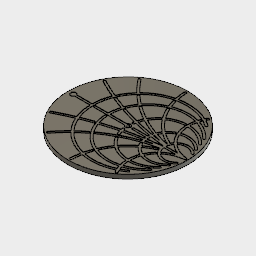
Resizable_Smith_Chart_Complete_7-18 (Autodesk Fusion 360 design; units mm, degrees)
Autodesk Fusion 360 part; units mm, degrees
note: some values were not read from the file. Set by a fixed rule: which sketch regions a step uses.
cylinder "CylinderPrimitive1" add diameter 355.6 height 12.7 placed x (1, 0, 0) y (0, 0, -1) z (0, 1, 0) at (0, 0, 0)
sketch "Smith Chart Overlay" plane through (0, 12.7, 0) normal (0, 1, 0) x (-1, 0, 0)
  circle A0 centre (0, 0) radius 177.8
  circle A1 centre (0, 0) radius 177.8
  line L0 (0, 0) -> (-177.8, 0)
  line L1 (0, 0) -> (-118.5333, 0) construction
  line L2 (0, 0) -> (-88.9, 0)
  line L3 (0, 0) -> (-59.2667, 0)
  circle A2 centre (-118.5333, 0) radius 59.2667 construction
  circle A3 centre (-88.9, 0) radius 88.9 construction
  circle A4 centre (-59.2667, 0) radius 118.5333 construction
  arc A5 (-106.68, -142.24) -> (-177.8, 0) centre (-177.8, -88.9) ccw construction
  line L4 (-177.8, 0) -> (-177.8, -88.9)
  line L5 (-177.8, 0) -> (-177.8, 88.9)
  line L6 (-177.8, 177.8) -> (-177.8, 0)
  line L7 (-177.8, 0) -> (-177.8, -177.8)
  line L8 (-177.8, 0) -> (-177.8, -355.6)
  arc A6 (-177.8, 0) -> (-106.68, 142.24) centre (-177.8, 88.9) ccw construction
  arc A7 (0, -177.8) -> (-177.8, 0) centre (-177.8, -177.8) ccw construction
  arc A8 (-177.8, 0) -> (0, 177.8) centre (-177.8, 177.8) ccw construction
  line L9 (-177.8, 355.6) -> (-177.8, 0)
  arc A9 (106.68, -142.24) -> (-177.8, 0) centre (-177.8, -355.6) ccw construction
  arc A10 (-177.8, 0) -> (106.68, 142.24) centre (-177.8, 355.6) ccw construction
  line L10 (-13.7583, 0) -> (-73.025, 0)
  line L11 (0, 0) -> (-59.2667, 0)
  line L12 (0, 0) -> (-35.56, 0)
  circle A11 centre (-35.56, 0) radius 142.24 construction
  line L13 (-177.8, 0) -> (-177.8, -711.2)
  arc A12 (156.8824, -83.6706) -> (-177.8, 0) centre (-177.8, -711.2) ccw construction
  arc A13 (-177.8, 0) -> (156.8824, 83.6706) centre (-177.8, 711.2) ccw construction
  line L14 (0, 0) -> (-142.24, 0) construction
  circle A14 centre (-142.24, 0) radius 35.56 construction
  line L15 (-35.56, 0) -> (177.8, 0) construction
  line L16 (-142.24, 0) -> (-168.4576, 24.024) construction
  line L17 (-142.24, 0) -> (-152.4, 0) construction
  line L18 (-142.24, 0) -> (-168.4576, -24.024) construction
  line L19 (-142.24, 0) -> (-168.4576, 24.024) construction
  line L20 (-118.5333, 0) -> (-162.2293, 40.04) construction
  line L21 (-118.5333, 0) -> (-149.1382, 0) construction
  arc A15 (-162.2293, -40.04) -> (-162.2293, 40.04) centre (-118.5333, 0) ccw construction
  line L22 (-118.5333, 0) -> (-162.2293, -40.04) construction
  line L23 (-118.5333, 0) -> (-162.2293, 40.04) construction
  line L24 (-88.9, 0) -> (-154.444, -60.06) construction
  line L25 (-88.9, 0) -> (-123.6401, 0) construction
  arc A16 (-154.444, -60.06) -> (-154.444, 60.06) centre (-88.9, 0) ccw construction
  line L26 (-88.9, 0) -> (-154.444, -60.06) construction
  line L27 (-88.9, 0) -> (-154.444, 60.06) construction
  line L28 (-35.56, 0) -> (-117.1455, -116.5162) construction
  line L29 (-35.56, 0) -> (214.1255, 0) construction
  line L30 (-59.2667, 0) -> (59.2667, 0) construction
  arc A17 (52.8595, 38.4432) -> (-92.456, 113.792) centre (-59.2667, 0) ccw
  line L31 (-177.8, -711.2) -> (-177.8, 711.2)
  line L32 (-59.2667, 0) -> (-146.6586, 80.08) construction
  line L33 (-59.2667, 0) -> (75.6719, 0) construction
  arc A18 (-146.6586, -80.08) -> (-146.6586, 80.08) centre (-59.2667, 0) ccw construction
  line L34 (-59.2667, 0) -> (-146.6586, -80.08) construction
  line L35 (-59.2667, 0) -> (-146.6586, 80.08) construction
  arc A19 (-117.1455, -116.5162) -> (-117.1455, 116.5162) centre (-35.56, 0) ccw construction
  line L36 (-35.56, 0) -> (-117.1455, -116.5162) construction
  line L37 (-35.56, 0) -> (-117.1455, 116.5162) construction
  arc A20 (-92.456, 113.792) -> (-97.8899, 127.8562) centre (-177.8, 88.9) ccw
  arc A21 (-60.0841, 9.8097) -> (52.8595, 38.4432) centre (-177.8, 711.2) ccw
  arc A22 (-60.0841, 9.8097) -> (-62.4703, 19.2216) centre (-118.5333, 0) ccw
  arc A23 (-107.3842, 7.0416) -> (-62.4703, 19.2216) centre (-177.8, 355.6) ccw
  arc A24 (-97.8899, -127.8562) -> (106.68, 0) centre (-35.56, 0) ccw
  arc A25 (-95.7385, -54.7077) -> (-116.4897, -24.5241) centre (-177.8, -88.9) ccw
  arc A26 (-92.456, -113.792) -> (-95.7385, -54.7077) centre (-177.8, -88.9) ccw
  arc A27 (-92.456, -113.792) -> (59.2667, 0) centre (-59.2667, 0) ccw
  circle A28 centre (106.68, 0) radius 7.62 construction
  circle A29 centre (59.2667, 0) radius 7.62 construction
  circle A30 centre (52.8595, -38.4432) radius 7.62 construction
  circle A31 centre (95.7385, -54.7077) radius 7.62 construction
  circle A32 centre (67.4414, -98.0966) radius 7.62 construction
  circle A33 centre (35.56, -71.12) radius 7.62 construction
  circle A34 centre (52.8595, 38.4432) radius 7.62 construction
  circle A35 centre (95.7385, 54.7077) radius 7.62 construction
  circle A36 centre (67.4414, 98.0966) radius 7.62 construction
  circle A37 centre (-97.8899, 127.8562) radius 7.62 construction
  circle A38 centre (-88.9, 88.9) radius 7.62 construction
  circle A39 centre (-13.6769, 109.4154) radius 7.62 construction
  circle A40 centre (-92.456, 113.792) radius 7.62 construction
  circle A41 centre (35.56, 71.12) radius 7.62 construction
  circle A42 centre (-2.7354, 21.8831) radius 7.62 construction
  circle A43 centre (-10.4588, 41.8353) radius 7.62 construction
  circle A44 centre (-35.56, 71.12) radius 7.62 construction
  circle A45 centre (0, 0) radius 15.24 construction
  circle A46 centre (-2.7354, -21.8831) radius 7.62 construction
  circle A47 centre (-10.4588, -41.8353) radius 7.62 construction
  circle A48 centre (-35.56, -71.12) radius 7.62 construction
  circle A49 centre (-88.9, -88.9) radius 7.62 construction
  circle A50 centre (-95.7385, -54.7077) radius 7.62 construction
  circle A51 centre (-95.7385, 54.7077) radius 7.62 construction
  circle A52 centre (-59.2667, 0) radius 7.62 construction
  circle A53 centre (-116.4897, -24.5241) radius 7.62 construction
  circle A54 centre (-116.4897, 24.5241) radius 7.62 construction
  circle A55 centre (-71.12, 35.56) radius 7.62 construction
  circle A56 centre (-4.3366, 138.7707) radius 7.62 construction
  circle A57 centre (-71.12, -35.56) radius 7.62 construction
  circle A58 centre (-92.456, -113.792) radius 7.62 construction
  circle A59 centre (-13.6769, -109.4154) radius 7.62 construction
  circle A60 centre (-97.8899, -127.8562) radius 7.62 construction
  circle A61 centre (-4.3366, -138.7707) radius 7.62 construction
  circle A62 centre (156.8824, -83.6706) radius 7.62 construction
  circle A63 centre (106.68, -142.24) radius 7.62 construction
  circle A64 centre (0, -177.8) radius 7.62 construction
  circle A65 centre (-106.68, -142.24) radius 7.62 construction
  circle A66 centre (-106.68, 142.24) radius 7.62 construction
  circle A67 centre (0, 177.8) radius 7.62 construction
  circle A68 centre (106.68, 142.24) radius 7.62 construction
  circle A69 centre (156.8824, 83.6706) radius 7.62 construction
  circle A70 centre (177.8, 0) radius 15.24 construction
  arc A71 (-117.1455, -116.5162) -> (-117.1455, 116.5162) centre (-35.56, 0) ccw
  line L38 (106.68, 0) -> (162.56, 0)
  arc A72 (150.1397, -80.1208) -> (95.7385, -54.7077) centre (-177.8, -711.2) ccw
  arc A73 (102.0429, -136.1933) -> (67.4414, -98.0966) centre (-177.8, -355.6) ccw
  arc A74 (-0.1633, -170.1817) -> (-4.3366, -138.7707) centre (-177.8, -177.8) ccw
  arc A75 (-102.3735, -135.9537) -> (-97.8899, -127.8562) centre (-177.8, -88.9) ccw
  arc A76 (95.7385, 54.7077) -> (150.1397, 80.1208) centre (-177.8, 711.2) ccw
  arc A77 (67.4414, 98.0966) -> (102.0429, 136.1933) centre (-177.8, 355.6) ccw
  arc A78 (-4.3366, 138.7707) -> (-0.1633, 170.1817) centre (-177.8, 177.8) ccw
  arc A79 (-97.8899, 127.8562) -> (-102.3735, 135.9537) centre (-177.8, 88.9) ccw
  arc A80 (-146.6586, -80.08) -> (-92.456, -113.792) centre (-59.2667, 0) ccw
  arc A81 (-111.202, 30.011) -> (-92.456, 113.792) centre (-177.8, 88.9) ccw
  arc A82 (-94.8474, -120.8699) -> (-92.456, -113.792) centre (-177.8, -88.9) ccw
  arc A83 (-6.1682, -131.3741) -> (-13.6769, -109.4154) centre (-177.8, -177.8) ccw
  arc A84 (61.8675, -92.9008) -> (35.56, -71.12) centre (-177.8, -355.6) ccw
  arc A85 (88.689, -51.8146) -> (52.8595, -38.4432) centre (-177.8, -711.2) ccw
  arc A86 (-168.4576, -24.024) -> (-168.4576, 24.024) centre (-142.24, 0) ccw
  arc A87 (-16.7577, -102.446) -> (-109.4154, -13.6769) centre (-177.8, -177.8) ccw
  arc A88 (-88.9076, -51.3308) -> (-60.0841, 9.8097) centre (-118.5333, 0) ccw
  circle A89 centre (-62.4703, 19.2216) radius 7.62 construction
  arc A90 (-62.4703, 19.2216) -> (29.4154, 66.6136) centre (-177.8, 355.6) ccw
  arc A91 (60.0542, 40.9532) -> (95.7385, 54.7077) centre (-177.8, 711.2) ccw
  arc A92 (41.6067, 75.7571) -> (67.4414, 98.0966) centre (-177.8, 355.6) ccw
  arc A93 (-10.8976, 116.5104) -> (-4.3366, 138.7707) centre (-177.8, 177.8) ccw
  line L39 (59.2667, 0) -> (0, 0)
  arc A94 (-1.3063, 15.1839) -> (-2.7354, 21.8831) centre (-88.9, 0) ccw
  arc A95 (59.0217, 7.6161) -> (52.8595, 38.4432) centre (-59.2667, 0) ccw
  line L40 (99.06, 0) -> (59.2667, 0)
  arc A96 (-95.7385, 54.7077) -> (-162.2293, 40.04) centre (-118.5333, 0) ccw
  circle A97 centre (-109.4154, 13.6769) radius 7.62 construction
  arc A98 (-102.446, 16.7577) -> (-13.6769, 109.4154) centre (-177.8, 177.8) ccw
  arc A99 (29.4154, -66.6136) -> (-107.3842, -7.0416) centre (-177.8, -355.6) ccw
  arc A100 (-81.287, -88.5734) -> (-1.3063, -15.1839) centre (-88.9, 0) ccw
  arc A101 (-154.444, -60.06) -> (-88.9, -88.9) centre (-88.9, 0) ccw
  line L41 (-15.24, 0) -> (-59.2667, 0)
  arc A102 (-60.0841, 9.8097) -> (-2.7354, 21.8831) centre (-177.8, 711.2) ccw
  arc A103 (-106.8574, 3.5471) -> (-60.0841, 9.8097) centre (-177.8, 711.2) ccw
  arc A104 (45.6382, -36.0105) -> (-106.8574, -3.5471) centre (-177.8, -711.2) ccw
  arc A105 (-88.9, 88.9) -> (-154.444, 60.06) centre (-88.9, 0) ccw
  arc A106 (-92.456, 113.792) -> (-146.6586, 80.08) centre (-59.2667, 0) ccw
  arc A107 (-65.3999, 26.2559) -> (-95.7385, 54.7077) centre (-118.5333, 0) ccw
  arc A108 (-14.3296, 48.399) -> (-88.9, 88.9) centre (-88.9, 0) ccw
  arc A109 (-2.7354, 21.8831) -> (-7.1644, 34.9643) centre (-88.9, 0) ccw
  circle A110 centre (0, 0) radius 7.62
  circle A111 centre (162.56, 0) radius 7.62
  circle A112 centre (150.1397, 80.1208) radius 3.175
  circle A113 centre (102.0429, 136.1933) radius 3.175
  circle A114 centre (-0.1633, 170.1817) radius 3.175
  circle A115 centre (-102.3735, 135.9537) radius 3.175
  circle A116 centre (150.1397, -80.1208) radius 3.175
  circle A117 centre (102.0429, -136.1933) radius 3.175
  circle A118 centre (-0.1633, -170.1817) radius 3.175
  circle A119 centre (-102.3735, -135.9537) radius 3.175
  circle A120 centre (-117.1455, -116.5162) radius 3.175
  circle A121 centre (-146.6586, -80.08) radius 3.175
  circle A122 centre (-154.444, -60.06) radius 3.175
  circle A123 centre (-168.4576, -24.024) radius 3.175
  circle A124 centre (-168.4576, 24.024) radius 3.175
  circle A125 centre (-162.2293, 40.04) radius 3.175
  circle A126 centre (-154.444, 60.06) radius 3.175
  circle A127 centre (-146.6586, 80.08) radius 3.175
  circle A128 centre (-117.1455, 116.5162) radius 3.175
  circle A129 centre (-14.3296, 48.399) radius 3.175
  circle A130 centre (-7.1644, 34.9643) radius 3.175
  circle A131 centre (-1.3063, 15.1839) radius 3.175
  circle A132 centre (-1.3063, -15.1839) radius 3.175
  circle A133 centre (-15.24, 0) radius 3.175
  circle A134 centre (59.0217, 7.6161) radius 3.175
  circle A135 centre (99.06, 0) radius 3.175
  circle A136 centre (60.0542, 40.9532) radius 3.175
  circle A137 centre (41.6067, 75.7571) radius 3.175
  circle A138 centre (-10.8976, 116.5104) radius 3.175
  circle A139 centre (-65.3999, 26.2559) radius 3.175
  circle A140 centre (-111.202, 30.011) radius 3.175
  circle A141 centre (-102.446, 16.7577) radius 3.175
  arc A142 (-162.2293, -40.04) -> (-95.7385, -54.7077) centre (-118.5333, 0) ccw
  circle A143 centre (-162.2293, -40.04) radius 3.175
  circle A144 centre (-88.9076, -51.3308) radius 3.175
  circle A145 centre (-81.287, -88.5734) radius 3.175
  circle A146 centre (45.6382, -36.0105) radius 3.175
  circle A147 centre (29.4154, -66.6136) radius 3.175
  circle A148 centre (-16.7577, -102.446) radius 3.175
  circle A149 centre (88.689, -51.8146) radius 3.175
  circle A150 centre (61.8675, -92.9008) radius 3.175
  circle A151 centre (-6.1682, -131.3741) radius 3.175
  circle A152 centre (-94.8474, -120.8699) radius 3.175
  circle A153 centre (29.4154, 66.6136) radius 3.175
  circle A154 centre (0, 0) radius 3.81
  circle A155 centre (-177.8, 0) radius 7.62 construction
  arc A156 (-170.187, 0.3266) -> (-116.4897, 24.5241) centre (-177.8, 88.9) ccw
  arc A157 (-116.4897, -24.5241) -> (-170.187, -0.3266) centre (-177.8, -88.9) ccw
  line L42 (-106.68, 0) -> (-170.18, 0)
  circle A158 centre (-170.18, 0) radius 3.501
  point P0 (-13.6769, 109.4154)
  point P1 (95.7385, 54.7077)
  point P2 (67.4414, 98.0966)
  point P3 (-97.8899, 127.8562)
  point P4 (106.68, 0)
  point P5 (95.7385, -54.7077)
  point P6 (67.4414, -98.0966)
  point P7 (-4.3366, -138.7707)
  point P8 (-97.8899, -127.8562)
  point P9 (-92.456, 113.792)
  point P10 (35.56, 71.12)
  point P11 (52.8595, 38.4432)
  point P12 (52.8595, -38.4432)
  point P13 (35.56, -71.12)
  point P14 (-13.6769, -109.4154)
  point P15 (-92.456, -113.792)
  point P16 (-35.56, 71.12)
  point P17 (-88.9, 88.9)
  point P18 (-10.4588, 41.8353)
  point P19 (-2.7354, -21.8831)
  point P20 (-88.9, -88.9)
  point P21 (-10.4588, -41.8353)
  point P22 (-35.56, -71.12)
  point P23 (-154.444, -60.06)
  point P24 (-2.7354, 21.8831)
  point P25 (-95.7385, 54.7077)
  point P26 (-71.12, 35.56)
  point P27 (-62.4703, 19.2216)
  point P28 (-60.0841, -9.8097)
  point P29 (-62.4703, -19.2216)
  point P30 (-71.12, -35.56)
  point P31 (-95.7385, -54.7077)
  point P32 (-60.0841, 9.8097)
  point P33 (-116.4897, 24.5241)
  point P34 (-177.8, 0)
  point P35 (-178.44, 0.0003)
  point P36 (106.68, 142.24)
  point P37 (0, 177.8)
  point P38 (156.8824, 83.6706)
  point P39 (156.8824, -83.6706)
  point P40 (177.8, 0)
  point P41 (106.68, -142.24)
  point P42 (0, -177.8)
  point P43 (59.2667, 0)
  point P44 (-177.8, -0.0001)
  point P45 (45.6382, 36.0105)
  point P46 (55.0978, 31.1594)
  point P47 (60.0542, 40.9532)
  point P48 (50.1577, 45.5682)
  point P49 (98.4798, 47.5979)
  point P50 (102.7565, 57.6761)
  point P51 (88.689, 51.8146)
  point P52 (92.6203, 61.6605)
  point P53 (99.06, 0)
  point P54 (106.4759, -7.6173)
  point P55 (106.4759, 7.6173)
  point P56 (59.0217, -7.6161)
  point P57 (51.6467, 0)
  point P58 (66.8867, 0)
  point P59 (88.689, -51.8146)
  point P60 (92.6203, -61.6605)
  point P61 (102.7565, -57.6761)
  point P62 (39.9337, -64.8802)
  point P63 (30.7944, -77.0659)
  point P64 (41.6067, -75.7571)
  point P65 (29.4154, -66.6136)
  point P66 (72.5469, -92.4398)
  point P67 (62.0403, -103.4717)
  point P68 (72.9027, -103.4105)
  point P69 (61.8675, -92.9008)
  point P70 (61.8675, 92.9008)
  point P71 (62.0403, 103.4717)
  point P72 (72.5469, 92.4398)
  point P73 (72.9027, 103.4105)
  point P74 (-10.8976, 116.5104)
  point P75 (-16.7577, 102.446)
  point P76 (-6.7409, 106.26)
  point P77 (-6.7409, 106.26)
  point P78 (-85.076, 115.6894)
  point P79 (-90.6379, 106.3921)
  point P80 (-94.9012, 121.009)
  point P81 (-99.6988, 111.4244)
  point P82 (-40.2616, 65.1234)
  point P83 (-31.1197, 77.3126)
  point P84 (-29.6655, 66.2909)
  point P85 (-41.8463, 75.4265)
  point P86 (-81.287, 88.5734)
  point P87 (-89.2266, 81.287)
  point P88 (-89.2266, 96.513)
  point P89 (-96.513, 88.5734)
  point P90 (-17.2204, 38.3217)
  point P91 (-7.1644, 34.9643)
  point P92 (-3.7741, 45.493)
  point P93 (-14.3296, 48.399)
  point P94 (114.3, 0)
  point P95 (98.4798, -47.5979)
  point P96 (59.0217, -7.6161)
  point P97 (60.0542, -40.9532)
  point P98 (50.1577, -45.5682)
  point P99 (45.6382, -36.0105)
  point P100 (55.0978, -31.1594)
  point P101 (-31.1197, -77.3126)
  point P102 (-41.8463, -75.4265)
  point P103 (-29.6655, -66.2909)
  point P104 (-40.2616, -65.1234)
  point P105 (-89.2266, -81.287)
  point P106 (-89.2266, -96.513)
  point P107 (-81.287, -88.5734)
  point P108 (-96.513, -88.5734)
  point P109 (-93.1118, -61.8607)
  point P110 (-98.968, -47.8059)
  point P111 (-102.9462, -57.1802)
  point P112 (-102.9462, -57.1802)
  point P113 (-111.8559, 18.4749)
  point P114 (-111.202, 30.011)
  point P115 (-122.3058, 29.4473)
  point P116 (-122.2277, 19.5103)
  point P117 (-98.968, 47.8059)
  point P118 (-102.9462, 57.1802)
  point P119 (-88.9076, 51.3308)
  point P120 (-93.1118, 61.8607)
  point P121 (-4.3366, 138.7707)
  point P122 (-66.9493, 29.1827)
  point P123 (-77.3126, 31.1197)
  point P124 (-76.0744, 41.3495)
  point P125 (-65.1234, 40.2616)
  point P126 (-104.6474, 124.3348)
  point P127 (-94.8474, 120.8699)
  point P128 (-101.5195, 134.5562)
  point P129 (-90.9535, 131.0106)
  point P130 (-17.2204, -38.3217)
  point P131 (-14.3296, -48.399)
  point P132 (-3.7741, -45.493)
  point P133 (-7.1644, -34.9643)
  point P134 (-4.9259, -29.1814)
  point P135 (4.64, -23.7983)
  point P136 (-1.1779, -14.4239)
  point P137 (-10.1309, -20.047)
  point P138 (-15.24, 0)
  point P139 (-1.3063, -15.1839)
  point P140 (15.24, 0)
  point P141 (-1.3063, 15.1839)
  point P142 (-1.1779, 14.4239)
  point P143 (4.64, 23.7983)
  point P144 (-10.1309, 20.047)
  point P145 (-4.9259, 29.1814)
  point P146 (3.0501, 136.8995)
  point P147 (-6.1682, 131.3741)
  point P148 (-11.8129, 140.2437)
  point P149 (-2.8236, 146.239)
  point P150 (-65.1234, -40.2616)
  point P151 (-76.0744, -41.3495)
  point P152 (-77.3126, -31.1197)
  point P153 (-51.6467, 0)
  point P154 (-59.7565, 7.6042)
  point P155 (-59.7565, 7.6042)
  point P156 (-66.8867, 0)
  point P157 (3.0501, -136.8995)
  point P158 (-2.8236, -146.239)
  point P159 (-6.1682, -131.3741)
  point P160 (-11.8129, -140.2437)
  point P161 (-20.8013, -112.1186)
  point P162 (-10.8976, -116.5104)
  point P163 (-6.7409, -106.26)
  point P164 (-16.7577, -102.446)
  point P165 (-192.3786, -267.9595)
  point P166 (-210, -290)
  point P167 (-225, -285)
  point P168 (-220, -260)
  point P169 (-180, -255)
  point P170 (-215, -245)
  point P171 (-185, -235)
  point P172 (-200, -225)
  point P173 (162.56, 0)
  point P174 (150.1397, 80.1208)
  point P175 (150.1397, -80.1208)
  point P176 (102.0429, -136.1933)
  point P177 (-0.1633, -170.1817)
  point P178 (-102.3735, -135.9537)
  point P179 (-102.3735, 135.9537)
  point P180 (-0.1633, 170.1817)
  point P181 (102.0429, 136.1933)
  point P182 (59.0217, 7.6161)
  point P183 (-104.6474, -124.3348)
  point P184 (-101.5195, -134.5562)
  point P185 (-90.9535, -131.0106)
  point P186 (-94.8474, -120.8699)
  point P187 (-88.9076, -51.3308)
  point P188 (-66.9493, -29.1827)
  point P189 (-122.2277, -19.5103)
  point P190 (-122.3058, -29.4473)
  point P191 (-111.202, -30.011)
  point P192 (-111.8559, -18.4749)
  point P193 (-109.4154, -13.6769)
  point P194 (-107.3842, -7.0416)
  point P195 (-60.4674, 11.8696)
  point P196 (-69.7044, 16.8276)
  point P197 (-65.3999, 26.2559)
  point P198 (-55.2891, 21.7701)
  point P199 (29.4154, 66.6136)
  point P200 (39.9337, 64.8802)
  point P201 (41.6067, 75.7571)
  point P202 (30.7944, 77.0659)
  point P203 (-109.4154, 13.6769)
  point P204 (-116.5104, 10.8976)
  point P205 (-107.2551, 6.3696)
  point P206 (-102.446, 16.7577)
  point P207 (-113.0829, 20.3563)
  point P208 (-106.8574, 3.5471)
  point P209 (-107.3842, 7.0416)
  point P210 (-106.8574, -3.5471)
  point P211 (-170.18, 0)
  point P212 (-170.187, 0.3266)
  point P213 (-170.187, -0.3266)
  point P214 (-106.68, 0)
  dimension "d6" = 355.6
  dimension "d7" = 177.8
  dimension "d8" = 118.5333
  dimension "d11" = 59.2667
  dimension "d12" = 118.5333
  dimension "d13" = 177.8
  dimension "d14" = 237.0667
  dimension "d15" = 88.9
  dimension "d17" = 88.9
  dimension "d18" = 88.9
  dimension "d19" = 177.8
  dimension "d20" = 177.8
  dimension "d21" = 355.6
  dimension "d22" = 88.9
  dimension "d23" = 177.8
  dimension "d24" = 355.6
  dimension "d25" = 59.2667
  dimension "d26" = 59.2667
  dimension "d31" = 35.56
  dimension "d32" = 284.48
  dimension "d33" = 711.2
  dimension "d34" = 711.2
  dimension "d35" = 142.24
  dimension "d36" = 71.12
  dimension "d54" = 137.5
  dimension "d55" = 85
  dimension "d56" = 137.5
  dimension "d57" = 85
  dimension "d58" = 137.5
  dimension "d59" = 85
  dimension "d60" = 125
  dimension "d64" = 118.5333
  dimension "d65" = 1422.4
  dimension "d68" = 137.5
  dimension "d69" = 85
  dimension "d70" = 110
  dimension "d79" = 15.24
  dimension "d80" = 15.24
  dimension "d81" = 15.24
  dimension "d82" = 15.24
  dimension "d83" = 15.24
  dimension "d84" = 15.24
  dimension "d85" = 15.24
  dimension "d86" = 15.24
  dimension "d87" = 15.24
  dimension "d88" = 15.24
  dimension "d89" = 15.24
  dimension "d90" = 15.24
  dimension "d91" = 15.24
  dimension "d92" = 15.24
  dimension "d93" = 15.24
  dimension "d94" = 15.24
  dimension "d95" = 15.24
  dimension "d96" = 30.48
  dimension "d97" = 15.24
  dimension "d98" = 15.24
  dimension "d99" = 15.24
  dimension "d100" = 15.24
  dimension "d101" = 15.24
  dimension "d102" = 15.24
  dimension "d103" = 15.24
  dimension "d104" = 15.24
  dimension "d105" = 15.24
  dimension "d106" = 15.24
  dimension "d107" = 15.24
  dimension "d108" = 15.24
  dimension "d109" = 15.24
  dimension "d110" = 15.24
  dimension "d111" = 15.24
  dimension "d112" = 15.24
  dimension "d113" = 15.24
  dimension "d114" = 15.24
  dimension "d115" = 15.24
  dimension "d116" = 15.24
  dimension "d117" = 15.24
  dimension "d118" = 15.24
  dimension "d119" = 15.24
  dimension "d120" = 15.24
  dimension "d121" = 30.48
  dimension "d251" = 15.24
  dimension "d288" = 15.24
  dimension "d341" = 15.24
  dimension "d342" = 15.24
  dimension "d348" = 6.35
  dimension "d349" = 6.35
  dimension "d350" = 6.35
  dimension "d351" = 6.35
  dimension "d352" = 6.35
  dimension "d353" = 6.35
  dimension "d354" = 6.35
  dimension "d355" = 6.35
  dimension "d356" = 6.35
  dimension "d357" = 6.35
  dimension "d358" = 6.35
  dimension "d359" = 6.35
  dimension "d360" = 6.35
  dimension "d361" = 6.35
  dimension "d362" = 6.35
  dimension "d363" = 6.35
  dimension "d364" = 6.35
  dimension "d365" = 6.35
  dimension "d366" = 6.35
  dimension "d367" = 6.35
  dimension "d368" = 6.35
  dimension "d369" = 6.35
  dimension "d370" = 6.35
  dimension "d371" = 6.35
  dimension "d372" = 6.35
  dimension "d373" = 6.35
  dimension "d374" = 6.35
  dimension "d375" = 6.35
  dimension "d376" = 6.35
  dimension "d377" = 6.35
  dimension "d382" = 6.35
  dimension "d383" = 6.35
  dimension "d384" = 6.35
  dimension "d385" = 6.35
  dimension "d386" = 6.35
  dimension "d387" = 6.35
  dimension "d388" = 6.35
  dimension "d389" = 6.35
  dimension "d390" = 6.35
  dimension "d391" = 6.35
  dimension "d405" = 6.35
  dimension "d412" = 7.62
  dimension "d416" = 15.24
  dimension "d429" = 7.002
  measures "d6" diameter of A1
  measures "d7" distance of A0.centre P34
  measures "d8" distance of A0.centre L1.end
  measures "d11" distance of A0.centre L3.end
  measures "d12" diameter of A2
  measures "d13" diameter of A3
  measures "d14" diameter of A4
  measures "d15" radius of A5
  measures "d17" distance of P34 A5.centre
  measures "d18" distance of P34 L5.end
  measures "d19" distance of L6.start P34
  measures "d20" distance of P34 L7.end
  measures "d21" distance of P34 L8.end
  measures "d22" radius of A6
  measures "d23" radius of A7
  measures "d24" distance of L9.start L0.end
  measures "d25" distance of L10.end L10.start
  measures "d26" distance of L3.end A0.centre
  measures "d31" distance of A0.centre L12.end
  measures "d32" diameter of A11
  measures "d33" distance of P34 L13.end
  measures "d34" distance of P34 A13.centre
  measures "d35" distance of A0.centre L14.end
  measures "d36" diameter of A14
  measures "d54" angle of L16 L17
  measures "d55" angle of L18 L19
  measures "d56" angle of L20 L21
  measures "d57" angle of L22 L23
  measures "d58" angle of L24 L25
  measures "d59" angle of L26 L27
  measures "d60" angle of L28 L29
  measures "d64" radius of A17
  measures "d65" distance of L13.end A13.centre
  measures "d68" angle of L32 L33
  measures "d69" angle of L34 L35
  measures "d70" angle of L36 L37
  measures "d79" diameter of A28
  measures "d80" diameter of A29
  measures "d81" diameter of A30
  measures "d82" diameter of A31
  measures "d83" diameter of A32
  measures "d84" diameter of A33
  measures "d85" diameter of A34
  measures "d86" diameter of A35
  measures "d87" diameter of A36
  measures "d88" diameter of A37
  measures "d89" diameter of A38
  measures "d90" diameter of A39
  measures "d91" diameter of A40
  measures "d92" diameter of A41
  measures "d93" diameter of A42
  measures "d94" diameter of A43
  measures "d95" diameter of A44
  measures "d96" diameter of A45
  measures "d97" diameter of A46
  measures "d98" diameter of A47
  measures "d99" diameter of A48
  measures "d100" diameter of A49
  measures "d101" diameter of A50
  measures "d102" diameter of A51
  measures "d103" diameter of A52
  measures "d104" diameter of A53
  measures "d105" diameter of A54
  measures "d106" diameter of A55
  measures "d107" diameter of A56
  measures "d108" diameter of A57
  measures "d109" diameter of A58
  measures "d110" diameter of A59
  measures "d111" diameter of A60
  measures "d112" diameter of A61
  measures "d113" diameter of A62
  measures "d114" diameter of A63
  measures "d115" diameter of A64
  measures "d116" diameter of A65
  measures "d117" diameter of A66
  measures "d118" diameter of A67
  measures "d119" diameter of A68
  measures "d120" diameter of A69
  measures "d121" diameter of A70
  measures "d251" diameter of A89
  measures "d288" diameter of A97
  measures "d341" diameter of A110
  measures "d342" diameter of A111
  measures "d348" diameter of A112
  measures "d349" diameter of A113
  measures "d350" diameter of A114
  measures "d351" diameter of A115
  measures "d352" diameter of A116
  measures "d353" diameter of A117
  measures "d354" diameter of A118
  measures "d355" diameter of A119
  measures "d356" diameter of A120
  measures "d357" diameter of A121
  measures "d358" diameter of A122
  measures "d359" diameter of A123
  measures "d360" diameter of A124
  measures "d361" diameter of A125
  measures "d362" diameter of A126
  measures "d363" diameter of A127
  measures "d364" diameter of A128
  measures "d365" diameter of A129
  measures "d366" diameter of A130
  measures "d367" diameter of A131
  measures "d368" diameter of A132
  measures "d369" diameter of A133
  measures "d370" diameter of A134
  measures "d371" diameter of A135
  measures "d372" diameter of A136
  measures "d373" diameter of A137
  measures "d374" diameter of A138
  measures "d375" diameter of A139
  measures "d376" diameter of A140
  measures "d377" diameter of A141
  measures "d382" diameter of A143
  measures "d383" diameter of A144
  measures "d384" diameter of A145
  measures "d385" diameter of A146
  measures "d386" diameter of A147
  measures "d387" diameter of A148
  measures "d388" diameter of A149
  measures "d389" diameter of A150
  measures "d390" diameter of A151
  measures "d391" diameter of A152
  measures "d405" diameter of A153
  measures "d412" diameter of A154
  measures "d416" diameter of A155
  measures "d429" diameter of A158
pipe "Pipe1" cut square section size 6.35 path "Smith Chart Overlay" along A71
pipe "Pipe2" cut square section size 6.35 path "Smith Chart Overlay" along A74
pipe "Pipe3" cut square section size 6.35 path "Smith Chart Overlay" along A72
pipe "Pipe4" cut square section size 6.35 path "Smith Chart Overlay" along L38
pipe "Pipe5" cut square section size 6.35 path "Smith Chart Overlay" along A76
pipe "Pipe6" cut square section size 6.35 path "Smith Chart Overlay" along A77
pipe "Pipe7" cut square section size 6.35 path "Smith Chart Overlay" along A78
pipe "Pipe8" cut square section size 6.35 path "Smith Chart Overlay" along A79
pipe "Pipe9" cut square section size 6.35 path "Smith Chart Overlay" along A75
pipe "Pipe10" cut square section size 6.35 path "Smith Chart Overlay" along A27
pipe "Pipe12" cut square section size 6.35 path "Smith Chart Overlay" along A26
pipe "Pipe13" cut square section size 6.35 path "Smith Chart Overlay" along A21
pipe "Pipe14" cut square section size 6.35 path "Smith Chart Overlay" along A17
pipe "Pipe15" cut square section size 6.35 path "Smith Chart Overlay" along A20
pipe "Pipe16" cut square section size 6.35 path "Smith Chart Overlay" along A22
pipe "Pipe21" cut square section size 6.35 path "Smith Chart Overlay" along A81
pipe "Pipe22" cut square section size 6.35 path "Smith Chart Overlay" along A82
pipe "Pipe23" cut square section size 6.35 path "Smith Chart Overlay" along A83
pipe "Pipe24" cut square section size 6.35 path "Smith Chart Overlay" along A84
pipe "Pipe25" cut square section size 6.35 path "Smith Chart Overlay" along A85
pipe "Pipe17" cut square section size 6.35 path "Smith Chart Overlay" along A23
pipe "Pipe27" cut square section size 6.35 path "Smith Chart Overlay" along A25
pipe "Pipe28" cut square section size 6.35 path "Smith Chart Overlay" along A80
pipe "Pipe29" cut square section size 6.35 path "Smith Chart Overlay" along A86
pipe "Pipe30" cut square section size 6.35 path "Smith Chart Overlay" along A87
pipe "Pipe31" cut square section size 6.35 path "Smith Chart Overlay" along A88
pipe "Pipe33" cut square section size 6.35 path "Smith Chart Overlay" along A90
pipe "Pipe34" cut square section size 6.35 path "Smith Chart Overlay" along A91
pipe "Pipe35" cut square section size 6.35 path "Smith Chart Overlay" along A92
pipe "Pipe36" cut square section size 6.35 path "Smith Chart Overlay" along A93
pipe "Pipe37" cut square section size 6.35 path "Smith Chart Overlay" along L39
pipe "Pipe38" cut square section size 6.35 path "Smith Chart Overlay" along A94
pipe "Pipe39" cut square section size 6.35 path "Smith Chart Overlay" along A95
pipe "Pipe40" cut square section size 6.35 path "Smith Chart Overlay" along L40
pipe "Pipe41" cut square section size 6.35 path "Smith Chart Overlay" along A96
pipe "Pipe42" cut square section size 6.35 path "Smith Chart Overlay" along A98
pipe "Pipe43" cut square section size 6.35 path "Smith Chart Overlay" along A99
pipe "Pipe44" cut square section size 6.35 path "Smith Chart Overlay" along A100
pipe "Pipe45" cut square section size 6.35 path "Smith Chart Overlay" along A101
pipe "Pipe46" cut square section size 6.35 path "Smith Chart Overlay" along L41
pipe "Pipe47" cut square section size 6.35 path "Smith Chart Overlay" along A103
pipe "Pipe48" cut square section size 6.35 path "Smith Chart Overlay" along A104
pipe "Pipe49" cut square section size 6.35 path "Smith Chart Overlay" along A105
pipe "Pipe50" cut square section size 6.35 path "Smith Chart Overlay" along A106
pipe "Pipe51" cut square section size 6.35 path "Smith Chart Overlay" along A107
pipe "Pipe52" cut square section size 6.35 path "Smith Chart Overlay" along A73
pipe "Pipe53" cut square section size 6.35 path "Smith Chart Overlay" along A108
pipe "Pipe54" cut square section size 6.35 path "Smith Chart Overlay" along A109
extrude "Extrude1" cut sketch "Smith Chart Overlay" against normal blind 3.175 contours A111
extrude "Extrude2" cut sketch "Smith Chart Overlay" against normal blind 3.175 contours L0 L2 L3 L11 L12 L39 A110 A154 | L0 L2 L3 L11 L12 L39 A110 A154 | L0 L2 L3 L11 L12 L39 A154 | L0 L2 L3 L11 L12 L39 A154
pipe "Pipe55" cut square section size 6.35 path "Smith Chart Overlay" along A142
extrude "Extrude3" cut sketch "Smith Chart Overlay" against normal blind 3.175 contours A112 | A113 | A114 | A115 | A116 | A117 | A118 | A119 | A120 | A128
extrude "Extrude4" cut sketch "Smith Chart Overlay" against normal blind 3.175 contours A121 | A127 | A134 | A135 | A136 | A137 | A138 | A146 | A147 | A148 | A149 | A150 | A151 | A152
extrude "Extrude5" cut sketch "Smith Chart Overlay" against normal blind 3.175 contours L0 L2 L3 L10 L11 L12 L41 A133 | L0 L2 L3 L10 L11 L12 L41 A133 | A122 | A126 | A129 | A130 | A131 | A132 | A145
extrude "Extrude6" cut sketch "Smith Chart Overlay" against normal blind 3.175 contours A125 | A139 | A143 | A144
extrude "Extrude7" cut sketch "Smith Chart Overlay" against normal blind 3.175 contours A123 | A125 | A140 | A141
extrude "Extrude8" cut sketch "Smith Chart Overlay" against normal blind 3.175 contours A123 | A124
extrude "Extrude9" cut sketch "Smith Chart Overlay" against normal blind 3.175 contours A153
extrude "Extrude10" add 1 faces at (0.2502, 9.525, 0.9264) along direction (0, 1, 0) blind 3.2
extrude "Extrude11" cut 1 faces at (0.2502, 12.725, 0.9264) along direction (0, -1, 0) blind 1.295
extrude "Extrude12" cut sketch "Smith Chart Overlay" against normal blind 1.397 contours L0 L2 L3 L11 L12 L39 A154 | L0 L2 L3 L11 L12 L39 A154
pipe "Pipe56" cut square section size 6.35 path "Smith Chart Overlay" along A157
pipe "Pipe57" cut square section size 6.35 path "Smith Chart Overlay" along A156
pipe "Pipe58" cut square section size 6.35 path "Smith Chart Overlay" along L42
extrude "Extrude13" cut sketch "Smith Chart Overlay" against normal blind 3.175 contours L0 L42 A158 | L0 L42 A158
extrude "Extrude14" add 1 faces at (154.0835, 9.525, 1.0583) along direction (0, 1, 0) blind 3.2
extrude "Extrude15" cut 1 faces at (154.0835, 12.725, 1.0583) along direction (0, -1, 0) blind 1.295
equation "body_diameter = 14 in"
equation "body_height = 0.5 in"
equation "d3 = body_height"
equation "d4 = body_diameter"
equation "d6 = body_diameter"
equation "d7 = radius"
equation "d8 = ( 2 * radius / ( radius + 2 * radius ) ) * radius"
equation "radius = body_diameter / 2"
equation "d10 = ( radius / ( radius + radius ) ) * radius"
equation "d11 = ( 0.5 * radius / ( radius + 0.5 * radius ) ) * radius"
equation "d12 = 2 * ( radius / ( radius + 2 * radius ) ) * radius"
equation "d13 = 2 * ( radius / ( radius + 1 * radius ) ) * radius"
equation "d14 = 2 * ( radius / ( radius + 0.5 * radius ) ) * radius"
equation "d15 = radius / ( 2 * radius ) * radius"
equation "d17 = radius / ( 2 * radius ) * radius"
equation "d18 = radius / ( 2 * radius ) * radius"
equation "d19 = radius / ( 1 * radius ) * radius"
equation "d20 = radius / ( 1 * radius ) * radius"
equation "d21 = radius / ( 0.5 * radius ) * radius"
equation "d22 = radius / ( 2 * radius ) * radius"
equation "d23 = radius / ( 1 * radius ) * radius"
equation "d24 = radius / ( 0.5 * radius ) * radius"
equation "d25 = ( 0.5 * radius / ( radius + 0.5 * radius ) ) * radius"
equation "d26 = ( 0.5 * radius / ( radius + 0.5 * radius ) ) * radius"
equation "d31 = ( 0.25 * radius / ( radius + 0.25 * radius ) ) * radius"
equation "d32 = 2 * ( radius / ( radius + 0.25 * radius ) ) * radius"
equation "d33 = radius / ( 0.25 * radius ) * radius"
equation "d34 = radius / ( 0.25 * radius ) * radius"
equation "d35 = ( 4 * radius / ( radius + 4 * radius ) ) * radius"
equation "d36 = 2 * ( radius / ( radius + 4 * radius ) ) * radius"
equation "arc_angle1 = 275 deg"
equation "arc_angle5 = 250 deg"
equation "arc_angle2 = 275 deg"
equation "arc_angle3 = 275 deg"
equation "arc_angle4 = 275 deg"
equation "d54 = arc_angle1 / 2"
equation "d55 = 360 deg - arc_angle1"
equation "d56 = arc_angle2 / 2"
equation "d57 = 360 deg - arc_angle2"
equation "d58 = arc_angle3 / 2"
equation "d59 = 360 deg - arc_angle3"
equation "d60 = arc_angle5 / 2"
equation "d64 = ( radius / ( radius + 0.5 * radius ) ) * radius"
equation "d65 = 2 * radius / ( 0.25 * radius ) * radius"
equation "d68 = arc_angle4 / 2"
equation "d69 = 360 deg - arc_angle4"
equation "d70 = 360 deg - arc_angle5"
equation "distance_guide = 0.3 in"
equation "distance_circle = 2 * distance_guide"
equation "d79 = distance_circle"
equation "d80 = distance_circle"
equation "d81 = distance_circle"
equation "d82 = distance_circle"
equation "d83 = distance_circle"
equation "d84 = distance_circle"
equation "d85 = distance_circle"
equation "d86 = distance_circle"
equation "d87 = distance_circle"
equation "d88 = distance_circle"
equation "d89 = distance_circle"
equation "d90 = distance_circle"
equation "d91 = distance_circle"
equation "d92 = distance_circle"
equation "d93 = distance_circle"
equation "d94 = distance_circle"
equation "d95 = distance_circle"
equation "d96 = 2 * distance_circle"
equation "d97 = distance_circle"
equation "d98 = distance_circle"
equation "d99 = distance_circle"
equation "d100 = distance_circle"
equation "d101 = distance_circle"
equation "d102 = distance_circle"
equation "d103 = distance_circle"
equation "d104 = distance_circle"
equation "d105 = distance_circle"
equation "d106 = distance_circle"
equation "d107 = distance_circle"
equation "d108 = distance_circle"
equation "d109 = distance_circle"
equation "d110 = distance_circle"
equation "d111 = distance_circle"
equation "d112 = distance_circle"
equation "d113 = distance_circle"
equation "d114 = distance_circle"
equation "d115 = distance_circle"
equation "d116 = distance_circle"
equation "d117 = distance_circle"
equation "d118 = distance_circle"
equation "d119 = distance_circle"
equation "d120 = distance_circle"
equation "d121 = 2 * distance_circle"
equation "trough_width = 0.25 in"
equation "d125 = trough_width"
equation "d129 = trough_width"
equation "d133 = trough_width"
equation "d137 = trough_width"
equation "d141 = trough_width"
equation "d145 = trough_width"
equation "d149 = trough_width"
equation "d153 = trough_width"
equation "d157 = trough_width"
equation "d161 = trough_width"
equation "d169 = trough_width"
equation "d173 = trough_width"
equation "d177 = trough_width"
equation "d181 = trough_width"
equation "d185 = trough_width"
equation "d189 = trough_width"
equation "d205 = trough_width"
equation "d209 = trough_width"
equation "d213 = trough_width"
equation "d217 = trough_width"
equation "d221 = trough_width"
equation "d229 = trough_width"
equation "d233 = trough_width"
equation "d237 = trough_width"
equation "d241 = trough_width"
equation "d245 = trough_width"
equation "d251 = distance_circle"
equation "d254 = trough_width"
equation "d258 = trough_width"
equation "d262 = trough_width"
equation "d266 = trough_width"
equation "d270 = trough_width"
equation "d274 = trough_width"
equation "d278 = trough_width"
equation "d282 = trough_width"
equation "d286 = trough_width"
equation "d288 = distance_circle"
equation "d291 = trough_width"
equation "d295 = trough_width"
equation "d299 = trough_width"
equation "d303 = trough_width"
equation "d307 = trough_width"
equation "d311 = trough_width"
equation "d315 = trough_width"
equation "d319 = trough_width"
equation "d323 = trough_width"
equation "d327 = trough_width"
equation "d331 = trough_width"
equation "d335 = trough_width"
equation "d339 = trough_width"
equation "d341 = distance_circle"
equation "d342 = distance_circle"
equation "trough_depth = 0.05 in"
equation "d344 = -trough_width / 2"
equation "d346 = -trough_width / 2"
equation "d348 = trough_width"
equation "d349 = trough_width"
equation "d350 = trough_width"
equation "d351 = trough_width"
equation "d352 = trough_width"
equation "d353 = trough_width"
equation "d354 = trough_width"
equation "d355 = trough_width"
equation "d356 = trough_width"
equation "d357 = trough_width"
equation "d358 = trough_width"
equation "d359 = trough_width"
equation "d360 = trough_width"
equation "d361 = trough_width"
equation "d362 = trough_width"
equation "d363 = trough_width"
equation "d364 = trough_width"
equation "d365 = trough_width"
equation "d366 = trough_width"
equation "d367 = trough_width"
equation "d368 = trough_width"
equation "d369 = trough_width"
equation "d370 = trough_width"
equation "d371 = trough_width"
equation "d372 = trough_width"
equation "d373 = trough_width"
equation "d374 = trough_width"
equation "d375 = trough_width"
equation "d376 = trough_width"
equation "d377 = trough_width"
equation "d380 = trough_width"
equation "d382 = trough_width"
equation "d383 = trough_width"
equation "d384 = trough_width"
equation "d385 = trough_width"
equation "d386 = trough_width"
equation "d387 = trough_width"
equation "d388 = trough_width"
equation "d389 = trough_width"
equation "d390 = trough_width"
equation "d391 = trough_width"
equation "d392 = -trough_width / 2"
equation "d394 = -trough_width / 2"
equation "d396 = -trough_width / 2"
equation "d398 = -trough_width / 2"
equation "d400 = -trough_width / 2"
equation "d402 = -trough_width / 2"
equation "d405 = trough_width"
equation "d406 = -trough_width / 2"
equation "d410 = -0.025 mm - trough_depth"
equation "d412 = 0.5 * distance_circle"
equation "end_hole_depth = 0.005 in"
equation "d414 = -end_hole_depth - trough_depth"
equation "d416 = distance_circle"
equation "d419 = trough_width"
equation "d423 = trough_width"
equation "d427 = trough_width"
equation "d429 = 1.1026771654 * trough_width"
equation "d430 = -trough_width / 2"
equation "d434 = -trough_depth - 0.025 mm"
